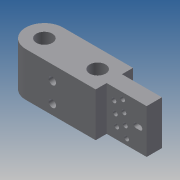
# Autodesk Inventor part: distal arm end
Saved by Autodesk Inventor 2013 (Build 170138000, 138)
## iProperties
Created: 2017-04-06
Part Number: distal arm end
Material: Generic
Document SubType Name: Modeling
Designer: employee
Density: 1 g/cm^3
Author: employee
Autodesk Inventor part; units mm, degrees
ref_plane "YZ Plane" through (0, 0, 0) normal (1, 0, 0) x (0, 1, 0)
ref_plane "XZ Plane" through (0, 0, 0) normal (0, 1, 0) x (-1, 0, 0)
ref_plane "XY Plane" through (0, 0, 0) normal (0, 0, 1) x (1, 0, 0)
sketch "Sketch1" plane through (0, 0, 0) normal (0, 0, 1) x (1, 0, 0)
  line L0 (0, 14) -> (52.5, 14)
  line L1 (52.5, 14) -> (52.5, 5.75)
  line L2 (52.5, 5.75) -> (82.5, 5.75)
  line L3 (82.5, 5.75) -> (82.5, -5.75)
  line L4 (82.5, -5.75) -> (52.5, -5.75)
  line L5 (52.5, -5.75) -> (52.5, -14)
  line L6 (52.5, -14) -> (0, -14)
  arc A0 (0, 14) -> (0, -14) centre (0, 0) ccw
  dimension "d0" = 82.5
  dimension "d1" = 30
  dimension "d2" = 14
  dimension "d3" = 11.5
  constraints: 14 end point, 4 parallel, 2 equal length, 2 point on circle, 2 tangent, 1 centre point, 1 coincident, 1 horizontal, 1 perpendicular, 1 vertical
  measures "d0" distance from line of L3 point (0, 0)
  measures "d1" distance of L3.end L4.end
  measures "d2" radius of A0
  measures "d3" distance of L2.end L3.end
extrude "Extrusion1" add sketch "Sketch1" along normal blind 33
sketch "Sketch2" plane through (0, 0, 0) normal (0, 0, -1) x (-1, 0, 0)
  arc A0 (0, -14) -> (0, 14) centre (0, 0) ccw projected
  circle A1 centre (0, 0) radius 6
  circle A2 centre (-40, 0) radius 6
  dimension "d6" = 12
  dimension "d8" = 40
  constraints: 2 centre point, 1 coincident, 1 equal radius, 1 horizontal alignment
  measures "d6" diameter of A2
  measures "d8" distance of A0.centre A2.centre
extrude "Extrusion2" cut sketch "Sketch2" against normal through all
sketch "Sketch3" plane through (52.5, -5.75, 0) normal (0, -1, 0) x (1, 0, 0)
  line L0 (30, 0) -> (30, 33) projected
  line L1 (0, 0) -> (0, 33) projected
  line L2 (25, 18.25) -> (22, 18.25)
  arc A0 (22, 18.25) -> (22, 14.75) centre (22, 16.5) ccw
  line L3 (22, 14.75) -> (25, 14.75)
  arc A1 (25, 14.75) -> (25, 18.25) centre (25, 16.5) ccw
  point P0 (-52.5, 0)
  point P1 (30, 16.5)
  dimension "d11" = 3
  dimension "d13" = 5
  dimension "d14" = 1.75
  constraints: 4 end point, 4 point on circle, 4 tangent, 2 centre point, 1 horizontal alignment, 1 midpoint, 1 parallel, 1 perpendicular
  measures "d11" distance of L3.start L3.end
  measures "d13" distance from line of A1.centre L0
  measures "d14" radius of A1
extrude "Extrusion3" cut sketch "Sketch3" against normal through all
sketch "Sketch4" plane through (52.5, -5.75, 0) normal (0, -1, 0) x (1, 0, 0)
  line L0 (0, 0) -> (0, 33) projected
  line L1 (5, 8.5) -> (5, 16.5) construction
  line L2 (5, 16.5) -> (5, 24.5) construction
  line L3 (12, 28.5) -> (12, 20.5) construction
  line L4 (12, 20.5) -> (12, 12.5) construction
  line L5 (12, 12.5) -> (12, 4.5) construction
  circle A0 centre (5, 8.5) radius 1.75 construction
  circle A1 centre (5, 16.5) radius 1.75 construction
  circle A2 centre (5, 24.5) radius 1.75 construction
  circle A3 centre (12, 28.5) radius 1.75
  circle A4 centre (12, 20.5) radius 1.75 construction
  circle A5 centre (12, 12.5) radius 1.75 construction
  circle A6 centre (12, 4.5) radius 1.75 construction
  line L6 (0, 0) -> (0, 33) projected
  circle A7 centre (5.5, 24.5) radius 1.75
  circle A8 centre (13, 20.5) radius 1.75
  circle A9 centre (6.5, 16.5) radius 1.75
  circle A10 centre (14, 12.5) radius 1.75
  circle A11 centre (7.5, 8.5) radius 1.75
  circle A12 centre (15, 4.5) radius 1.75
  point P0 (-52.5, 0)
  point P1 (12, 16.5)
  point P2 (0, 16.5)
  dimension "d17" = 5
  dimension "d18" = 7
  dimension "d19" = 3.5
  dimension "d20" = 8
  dimension "d21" = 0.5
  dimension "d22" = 1
  dimension "d23" = 1.5
  dimension "d24" = 2
  dimension "d25" = 2.5
  dimension "d26" = 3
  constraints: 13 centre point, 12 equal radius, 10 end point, 8 horizontal alignment, 7 coincident, 4 equal length, 3 collinear, 2 midpoint, 2 parallel
  measures "d17" distance between parallel lines of L0 L2
  measures "d18" distance between parallel lines of L2 L3
  measures "d19" diameter of A2
  measures "d20" distance of L1.end L2.end
  measures "d21" distance of L2.end A7.centre
  measures "d22" distance of L3.end A8.centre
  measures "d23" distance of L1.end A9.centre
  measures "d24" distance of L4.end A10.centre
  measures "d25" distance of L1.start A11.centre
  measures "d26" distance of L5.end A12.centre
extrude "Extrusion4" cut sketch "Sketch4" against normal through all
sketch "Sketch5" plane through (0, -14, 0) normal (0, -1, 0) x (1, 0, 0)
  line L0 (52.5, 0) -> (0, 0) projected
  line L1 (0, 33) -> (52.5, 33) projected
  line L2 (0, 0) -> (0, 33) projected
  line L3 (43, -22.7639) -> (43, 127.2361)
  line L4 (37, -22.7639) -> (37, 127.2361)
  line L5 (37, 33) -> (43, 33)
  line L6 (40, 33) -> (40, 0)
  line L7 (0, 14.9) -> (40, 14.9)
  line L8 (20, 14.9) -> (20, 22.275)
  circle A0 centre (20, 22.275) radius 2.75
  line L9 (20, 14.9) -> (20, 7.525)
  circle A1 centre (20, 7.525) radius 2.75
  dimension "d32" = 18.1
  dimension "d34" = 7.375
  dimension "d35" = 5.5
  constraints: 14 end point, 7 point on line, 3 perpendicular, 2 centre point, 2 coincident, 2 collinear, 2 midpoint, 2 vertical, 1 equal radius, 4 other
  measures "d32" distance between parallel lines of L7 L1
  measures "d34" distance of L8.start L8.end
  measures "d35" diameter of A0
extrude "Extrusion5" cut sketch "Sketch5" against normal through all contours A1 | A0
sketch "Sketch6" plane through (0, 14, 0) normal (0, 1, 0) x (1, 0, 0)
  circle A0 centre (20, -22.275) radius 2.75 projected
  line L0 (22.3094, -18.275) -> (24.6188, -22.275)
  line L1 (24.6188, -22.275) -> (22.3094, -26.275)
  line L2 (22.3094, -26.275) -> (17.6906, -26.275)
  line L3 (17.6906, -26.275) -> (15.3812, -22.275)
  line L4 (15.3812, -22.275) -> (17.6906, -18.275)
  line L5 (17.6906, -18.275) -> (22.3094, -18.275)
  dimension "d38" = 8
  constraints: 12 end point, 1 coincident, 1 horizontal, 13 other
  measures "d38" distance between parallel lines of L2 L5
extrude "Extrusion6" cut sketch "Sketch6" against normal blind 5
sketch "Sketch7" plane through (0, -14, 0) normal (0, -1, 0) x (1, 0, 0)
  circle A0 centre (20, 7.525) radius 2.75 projected
  line L0 (17.6906, 11.525) -> (22.3094, 11.525)
  line L1 (22.3094, 11.525) -> (24.6188, 7.525)
  line L2 (24.6188, 7.525) -> (22.3094, 3.525)
  line L3 (22.3094, 3.525) -> (17.6906, 3.525)
  line L4 (17.6906, 3.525) -> (15.3812, 7.525)
  line L5 (15.3812, 7.525) -> (17.6906, 11.525)
  dimension "d41" = 8
  constraints: 12 end point, 1 coincident, 1 horizontal, 13 other
  measures "d41" distance between parallel lines of L3 L0
extrude "Extrusion7" cut sketch "Sketch7" against normal blind 5
sketch "Sketch8" plane through (0, 0, 33) normal (0, 0, 1) x (1, 0, 0)
  circle A0 centre (0, 0) radius 6 projected
  circle A1 centre (40, 0) radius 6 projected
  line L0 (0, 1.5) -> (40, 1.5)
  line L1 (40, 1.5) -> (40, -1.5)
  line L2 (40, -1.5) -> (0, -1.5)
  line L3 (0, -1.5) -> (0, 1.5)
  dimension "d44" = 3
  constraints: 8 end point, 2 coincident, 2 midpoint, 2 parallel, 1 horizontal, 1 perpendicular
  measures "d44" distance of L0.end L1.end
extrude "Extrusion8" cut sketch "Sketch8" against normal through all contours A0 L2 L3 L0 | A0 L0 A1 L2 | L0 L1 L2 A1 picked at (2, 0) picked at (38.0071, -0.1683)
body "Solid1"
